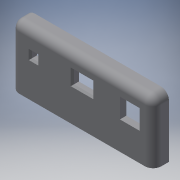
# Autodesk Inventor part: PIUIODaughterBoardCover
Saved by Autodesk Inventor 2016 (Build 200138000, 138)
## iProperties
Created: 2015-09-28
Part Number: PIUIODaughterBoardCover
Material: Generic
Document SubType Name: Modeling
Designer: Jake
Density: 1 g/cm^3
Appearance: Default
Author: Jake
Autodesk Inventor part; units mm, degrees
ref_plane "YZ Plane" through (0, 0, 0) normal (1, 0, 0) x (0, 1, 0)
ref_plane "XZ Plane" through (0, 0, 0) normal (0, 1, 0) x (-1, 0, 0)
ref_plane "XY Plane" through (0, 0, 0) normal (0, 0, 1) x (1, 0, 0)
sketch "Sketch1" plane through (0, 0, 0) normal (0, 0, 1) x (1, 0, 0)
  line L0 (0, 0) -> (50.8, 0)
  line L1 (50.8, 0) -> (50.8, 19.05)
  line L2 (50.8, 19.05) -> (0, 19.05)
  line L3 (0, 19.05) -> (0, 0)
  line L4 (0, 0) -> (0, -2.54)
  line L5 (0, -2.54) -> (-2.54, -2.54)
  line L6 (-2.54, -2.54) -> (-2.54, 19.05)
  line L7 (-2.54, 19.05) -> (-2.54, 21.59)
  line L8 (-2.54, 21.59) -> (53.34, 21.59)
  line L9 (53.34, 21.59) -> (53.34, -2.54)
  line L10 (53.34, -2.54) -> (0, -2.54)
  dimension "d0" = 50.8
  dimension "d1" = 19.05
  dimension "d2" = 50.8
  dimension "d3" = 2.54
  dimension "d4" = 2.54
  dimension "d5" = 2.54
  dimension "d6" = 55.88
  constraints: 22 end point, 6 perpendicular, 2 horizontal, 2 point on line
  measures "d0" distance of L0.start L0.end
  measures "d1" distance of L0.end L1.end
  measures "d2" distance of L1.end L2.end
  measures "d3" distance of L0.start L4.end
  measures "d4" distance of L4.end L5.end
  measures "d5" distance of L6.end L7.end
  measures "d6" distance of L7.end L8.end
extrude "Extrusion1" add sketch "Sketch1" along normal blind 1.905
sketch "Sketch2" plane through (0, 0, 1.905) normal (0, 0, 1) x (1, 0, 0)
  line L0 (-2.54, -2.54) -> (-2.54, 21.59)
  line L1 (-2.54, 21.59) -> (53.34, 21.59)
  line L2 (53.34, 21.59) -> (-2.54, 21.59) projected
  line L3 (53.34, 21.59) -> (53.34, -2.54)
  line L4 (53.34, -2.54) -> (-2.54, -2.54)
  line L5 (-2.54, -2.54) -> (53.34, -2.54) projected
  point P0 (0, 0)
  constraints: 8 end point, 2 collinear, 1 perpendicular, 1 vertical
extrude "Extrusion2" add sketch "Sketch2" along normal blind 2.54
sketch "Sketch3" plane through (0, 0, 0) normal (0, 0, -1) x (-1, 0, 0)
  line L0 (0, 0) -> (2.54, 0)
  line L1 (2.54, 21.59) -> (2.54, -2.54) projected
  line L2 (2.54, 0) -> (2.54, 19.05)
  line L3 (2.54, 0) -> (0.635, 0)
  line L4 (0.635, 0) -> (0.635, 19.05)
  line L5 (0.635, 19.05) -> (0, 19.05)
  line L6 (0, 19.05) -> (0, 0)
  line L7 (0, 0) -> (-50.8, 0) projected
  line L8 (0, 19.05) -> (0.635, 19.05)
  line L9 (-50.8, 0) -> (-51.435, 0)
  line L10 (-51.435, 0) -> (-51.435, 19.05)
  line L11 (-51.435, 19.05) -> (-50.8, 19.05)
  line L12 (-50.8, 19.05) -> (-50.8, 0)
  dimension "d11" = 1.905
  dimension "d12" = 0.635
  dimension "d13" = 19.05
  constraints: 22 end point, 5 point on line, 4 perpendicular, 2 horizontal, 1 parallel
  measures "d11" distance of L0.end L3.end
  measures "d12" distance of L7.end L9.end
  measures "d13" distance of L9.end L10.end
extrude "Extrusion3" cut sketch "Sketch3" against normal blind 1.905
sketch "Sketch4" plane through (0, 0, 0) normal (0, 0, -1) x (-1, 0, 0)
  line L0 (2.54, -2.54) -> (-53.34, -2.54) projected
  line L1 (0, 0) -> (-51.435, 0)
  line L2 (-51.435, 0) -> (-51.435, 19.05) projected
  line L3 (-51.435, 0) -> (-51.435, -2.54)
  line L4 (-51.435, -2.54) -> (0, -2.54)
  line L5 (0.635, 0) -> (0.635, -2.54)
  line L6 (0.635, 0) -> (0, 0)
  line L7 (0.635, 0) -> (-51.435, 0) projected
  line L8 (0.635, -2.54) -> (0, -2.54)
  constraints: 12 end point, 3 collinear, 3 perpendicular, 3 point on line
extrude "Extrusion4" cut sketch "Sketch4" against normal blind 1.905
sketch "Sketch5" plane through (0, 0, 4.445) normal (0, 0, 1) x (1, 0, 0)
  line L0 (-2.54, 21.59) -> (7.62, 21.59)
  line L1 (53.34, 21.59) -> (-2.54, 21.59) projected
  line L2 (7.62, 21.59) -> (7.62, 11.43)
  line L3 (-2.54, 21.59) -> (5.08, 21.59)
  line L4 (5.08, 21.59) -> (5.08, 13.97)
  line L5 (5.08, 13.97) -> (7.62, 13.97)
  line L6 (5.08, 13.97) -> (5.08, 11.43)
  line L7 (5.08, 11.43) -> (7.62, 11.43)
  line L8 (-2.54, 21.59) -> (26.67, 21.59)
  line L9 (-2.54, 21.59) -> (19.05, 21.59)
  line L10 (19.05, 10.795) -> (26.67, 10.795)
  line L11 (26.67, 18.415) -> (19.05, 18.415)
  line L12 (26.67, 21.59) -> (29.21, 21.59)
  line L13 (19.05, 21.59) -> (21.59, 21.59)
  line L14 (21.59, 10.795) -> (29.21, 10.795)
  line L15 (29.21, 10.795) -> (29.21, 21.59)
  line L16 (26.67, 18.415) -> (29.21, 18.415)
  line L17 (21.59, 21.59) -> (21.59, 18.415)
  line L18 (29.21, 18.415) -> (21.59, 18.415)
  line L19 (21.59, 18.415) -> (21.59, 10.795)
  line L20 (53.34, 21.59) -> (40.64, 21.59)
  line L21 (40.64, 21.59) -> (40.64, 8.89)
  line L22 (53.34, 21.59) -> (47.625, 21.59)
  line L23 (47.625, 21.59) -> (47.625, 15.875)
  line L24 (47.625, 15.875) -> (40.64, 15.875)
  line L25 (47.625, 15.875) -> (47.625, 8.89)
  line L26 (47.625, 8.89) -> (40.64, 8.89)
  point P0 (0, 0)
  dimension "d18" = 10.16
  dimension "d19" = 10.16
  dimension "d20" = 7.62
  dimension "d21" = 7.62
  dimension "d22" = 29.21
  dimension "d23" = 21.59
  dimension "d24" = 10.795
  dimension "d25" = 3.175
  dimension "d26" = 2.54
  dimension "d27" = 2.54
  dimension "d28" = 12.7
  dimension "d29" = 12.7
  dimension "d30" = 5.715
  constraints: 52 end point, 14 point on line, 11 perpendicular, 1 collinear, 1 horizontal, 1 vertical
  measures "d18" distance of L0.start L0.end
  measures "d19" distance of L0.end L2.end
  measures "d20" distance of L0.start L3.end
  measures "d21" distance of L3.end L4.end
  measures "d22" distance of L0.start L8.end
  measures "d23" distance of L0.start L9.end
  measures "d24" distance of L9.end L10.start
  measures "d25" distance of L8.end L11.start
  measures "d26" distance of L8.end L12.end
  measures "d27" distance of L9.end L13.end
  measures "d28" distance of L1.start L20.end
  measures "d29" distance of L20.end L21.end
  measures "d30" distance of L1.start L22.end
extrude "Extrusion5" cut sketch "Sketch5" against normal blind 2.54 contours L5 L2 L7 L6 | L25 L26 L21 L24 | L15 L14 L10 L19 L11 L16
move faces "Move1" translate (0, -2.54, 0) faces at (26.67, 18.415, 3.5983)
move faces "Move2" translate (0, 0, -0.635) faces at (34.0783, 20.7433, 0)
sketch "Sketch6" plane through (53.34, 21.59, -0.635) normal (0, 0, -1) x (-1, 0, 0)
  line L0 (1.905, -2.54) -> (1.905, -13.335)
  line L1 (1.905, -24.13) -> (1.905, -2.54) projected
  line L2 (1.905, -13.335) -> (1.905, -10.795)
  line L3 (1.905, -13.335) -> (1.905, -15.875)
  line L4 (1.905, -15.875) -> (3.175, -15.875)
  line L5 (3.175, -15.875) -> (3.175, -10.795)
  line L6 (3.175, -10.795) -> (1.905, -10.795)
  line L7 (1.905, -2.54) -> (27.94, -2.54)
  line L8 (1.905, -2.54) -> (53.975, -2.54) projected
  line L9 (27.94, -2.54) -> (30.48, -2.54)
  line L10 (27.94, -2.54) -> (25.4, -2.54)
  line L11 (25.4, -2.54) -> (25.4, -3.81)
  line L12 (25.4, -3.81) -> (30.48, -3.81)
  line L13 (30.48, -3.81) -> (30.48, -2.54)
  line L14 (53.975, -2.54) -> (53.975, -13.335)
  line L15 (53.975, -2.54) -> (53.975, -24.13) projected
  line L16 (53.975, -13.335) -> (53.975, -10.795)
  line L17 (53.975, -10.795) -> (52.705, -10.795)
  line L18 (52.705, -10.795) -> (52.705, -15.875)
  line L19 (52.705, -15.875) -> (53.975, -15.875)
  line L20 (53.975, -15.875) -> (53.975, -10.795)
  point P0 (53.34, -21.59)
  dimension "d39" = 10.795
  dimension "d40" = 2.54
  dimension "d41" = 2.54
  dimension "d42" = 5.08
  dimension "d43" = 26.035
  dimension "d44" = 2.54
  dimension "d45" = 2.54
  dimension "d46" = 1.27
  dimension "d47" = 5.08
  dimension "d48" = 10.795
  dimension "d49" = 2.54
  dimension "d51" = 1.27
  dimension "d52" = 5.08
  constraints: 36 end point, 6 perpendicular, 6 point on line, 3 midpoint, 1 collinear, 1 horizontal
  measures "d39" distance of L0.start L0.end
  measures "d40" distance of L0.end L2.end
  measures "d41" distance of L0.end L3.end
  measures "d42" distance of L4.end L5.end
  measures "d43" distance of L0.start L7.end
  measures "d44" distance of L7.end L9.end
  measures "d45" distance of L7.end L10.end
  measures "d46" distance of L10.end L11.end
  measures "d47" distance of L11.end L12.end
  measures "d48" distance of L8.end L14.end
  measures "d49" distance of L14.end L16.end
  measures "d51" distance of L16.end L17.end
  measures "d52" distance of L17.end L18.end
extrude "Extrusion6" add sketch "Sketch6" against normal blind 0.889
move faces "Move3" translate (0, 0, -0.381) faces at (26.2467, 20.7433, -0.635)
move faces "Move4" translate (0, 0, -0.762) faces at (24.5533, 20.7433, -1.016)
sketch "Sketch10" plane through (50.165, 10.795, 0.254) normal (0, 1, 0) x (1, 0, 0)
  line L0 (1.27, 2.032) -> (1.27, 0) projected
  line L1 (1.27, 2.032) -> (1.27, 0.762)
  line L2 (0, 2.032) -> (0, 0) projected
  line L3 (1.27, 0.762) -> (0, 2.032)
  line L4 (1.27, 0) -> (0, 0) projected
  line L5 (0, 2.032) -> (0, 0)
  line L6 (0, 0) -> (1.27, 0)
  line L7 (1.27, 0) -> (1.27, 0.762)
  point P0 (-50.165, 0.254)
  dimension "d70" = 1.27
  constraints: 10 end point, 2 perpendicular, 1 parallel, 1 point on line
  measures "d70" distance of L0.start L1.end
extrude "Extrusion10" cut sketch "Sketch10" against normal blind 25.4
sketch "Sketch11" plane through (22.86, 17.78, 0.254) normal (-1, 0, 0) x (0, 0, 1)
  line L0 (-2.032, 1.27) -> (-0.762, 1.27)
  line L1 (-2.032, 1.27) -> (0, 1.27) projected
  line L2 (-2.032, 0) -> (-2.032, 1.27) projected
  line L3 (-0.762, 1.27) -> (-2.032, 0)
  line L4 (-2.032, 0) -> (0, 0) projected
  line L5 (-2.032, 0) -> (0, 0)
  line L6 (0, 0) -> (0, 1.27)
  line L7 (0, 1.27) -> (-0.762, 1.27)
  point P0 (-0.254, -17.78)
  dimension "d73" = 1.27
  constraints: 10 end point, 2 perpendicular, 1 parallel, 1 point on line
  measures "d73" distance of L0.start L0.end
extrude "Extrusion11" cut sketch "Sketch11" against normal blind 6.35 contours L1 L6 L4 L3
sketch "Sketch12" plane through (-0.635, 5.715, 0.254) normal (0, -1, 0) x (1, 0, 0)
  line L0 (1.27, -2.032) -> (0, -2.032) projected
  line L1 (0, -2.032) -> (0, -0.762)
  line L2 (0, -2.032) -> (0, 0) projected
  line L3 (0, -0.762) -> (1.27, -2.032)
  line L4 (1.27, -2.032) -> (1.27, 0)
  line L5 (0, 0) -> (1.27, 0) projected
  line L6 (1.27, 0) -> (0, 0)
  line L7 (0, 0) -> (0, -0.762)
  point P0 (0.635, -0.254)
  dimension "d76" = 1.27
  constraints: 10 end point, 1 collinear, 1 parallel, 1 perpendicular, 1 point on line
  measures "d76" distance of L0.end L1.end
extrude "Extrusion12" cut sketch "Sketch12" against normal blind 6.35 contours L3 L2 L5 L4
sketch "Sketch13" plane through (0, 0, 4.445) normal (0, 0, 1) x (1, 0, 0)
  line L0 (53.34, -2.54) -> (53.34, 21.59) projected
  line L1 (53.34, 21.59) -> (44.1325, 21.59)
  line L2 (53.34, 21.59) -> (-2.54, 21.59) projected
  line L3 (44.1325, 21.59) -> (44.1325, 16.2433)
  line L4 (48.006, 12.3825) -> (48.006, 8.4963)
  line L5 (48.006, 8.4963) -> (40.259, 8.4963)
  line L6 (40.259, 8.4963) -> (40.259, 16.2433)
  line L7 (40.259, 16.2433) -> (48.006, 16.2433)
  line L8 (48.006, 16.2433) -> (48.006, 12.3825)
  point P0 (0, 0)
  dimension "d79" = 9.2075
  dimension "d82" = 3.8862
  dimension "d83" = 7.747
  dimension "d84" = 7.747
  dimension "d85" = 7.747
  constraints: 14 end point, 3 perpendicular, 2 point on line, 1 midpoint
  measures "d79" distance of L0.end L1.end
  measures "d82" distance of L4.start L4.end
  measures "d83" distance of L4.end L5.end
  measures "d84" distance of L5.end L6.end
  measures "d85" distance of L6.end L7.end
extrude "Extrusion13" cut sketch "Sketch13" against normal blind 6.35
fillet "Fillet1" radius 3.175 2 edges at (-2.54, 9.525, 4.445) (53.34, 9.525, 4.445)
fillet "Fillet2" radius 3.175 5 edges at (-1.6101, 21.59, 3.5151) (-2.54, 21.59, -0.254) (52.4101, 21.59, 3.5151) (53.34, 21.59, -0.254) (25.4, 21.59, 4.445)
chamfer "Chamfer1" distance 0.635 angle 45 8 edges at (25.4, 15.875, 4.445) (29.21, 13.335, 4.445) (25.4, 10.795, 4.445) (21.59, 13.335, 4.445) (6.35, 13.97, 4.445) (7.62, 12.7, 4.445) (6.35, 11.43, 4.445) (5.08, 12.7, 4.445)
body "Solid1"
